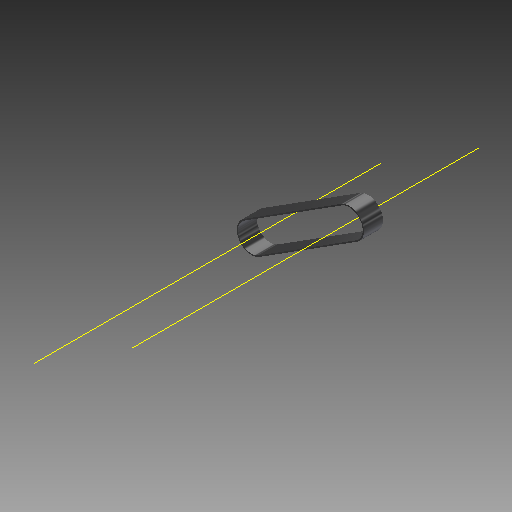
# Autodesk Inventor part: Synchronous Belt
Saved by Autodesk Inventor 2019.4 (Build 234330000, 330)
## iProperties
Created: 2020-01-17
Part Number: Synchronous Belt
Material: Rubber
Document SubType Name: Modeling
Designer: admin
Density: 1 g/cm^3
Appearance: Rubber - Black - Version 1.1
CustomPartVersion: 1
Author: admin
Autodesk Inventor part; units mm, degrees
sketch "Sketch Path" plane through (0, 0, 0) normal (0, 0, 1) x (1, 0, 0)
  arc A0 (-167.8042, 60.329) -> (-155.0122, 40.1722) centre (-161.4082, 50.2506) ccw
  arc A1 (-72.6903, 92.4153) -> (-85.4822, 112.5721) centre (-79.0862, 102.4937) ccw
  line L0 (-72.6903, 92.4153) -> (-155.0122, 40.1722)
  line L1 (-167.8042, 60.329) -> (-85.4822, 112.5721)
  constraints: 4 end point, 4 point on circle, 2 centre point
ref_plane "Cross Section Plane" through (-155.0122, 40.1722, 0) normal (0.844328, 0.5358266, 0) x (0, 0, 1)
ref_plane "Work Plane2" through (-161.4082, 50.2506, 0) normal (-1, 0, 0) x (0, 0, 1)
ref_plane "Work Plane3" through (-79.0862, 102.4937, 0) normal (-0.9781476, -0.2079117, 0) x (0, 0, 1)
sketch "Cross Section" plane through (-155.0122, 40.1722, 0) normal (0.844328, 0.5358266, 0) x (0, 0, 1)
  line L0 (-8, 0.5) -> (8, 0.5)
  line L1 (8, 0.5) -> (8, -0.5)
  line L2 (8, -0.5) -> (-8, -0.5)
  line L3 (-8, -0.5) -> (-8, 0.5)
  line L4 (-8, 0) -> (8, 0) construction
  point P0 (0, 0)
  point P1 (0, 0)
  dimension "d0" = 16
  dimension "d4" = 0.5
  dimension "d5" = 0.5
  constraints: 10 end point, 3 midpoint, 2 parallel, 1 coincident, 1 horizontal, 1 perpendicular, 1 other
  measures "d0" distance between parallel lines of L1 L3
  measures "d4" distance between parallel lines of L2 L4
  measures "d5" distance between parallel lines of L4 L0
sweep "Belt" add profiles "Cross Section" path "Sketch Path" path curves L1 A1 L0 A0
equation "\"d0\" = da_B"
equation "\"d4\" = da_a"
equation "\"d5\" = da_a2"
equation "\"da_B\" = 16"
equation "\"da_pb\" = 5"
equation "\"da_a\" = 0.5"
equation "\"da_S\" = 2.65"
equation "\"da_Beta\" = 20deg"
equation "\"da_Ht\" = 1.2"
equation "\"da_H\" = 2.2"
equation "\"da_a2\" = 0.5"
body "Solid1"
